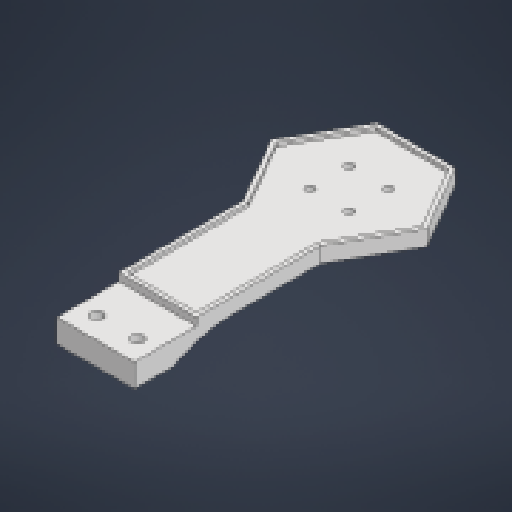
# Autodesk Inventor part: Arm
Saved by Autodesk Inventor 2023 (Build 270158000, 158)
## iProperties
Created: 2023-01-21
Part Number: Arm
Material: Generic
Document SubType Name: Modeling
Designer: Michael
Density: 1 g/cm^3
Appearance: Default
Author: Michael
Autodesk Inventor part; units mm, degrees
ref_plane "YZ Plane" through (0, 0, 0) normal (1, 0, 0) x (0, 1, 0)
ref_plane "XZ Plane" through (0, 0, 0) normal (0, 1, 0) x (-1, 0, 0)
ref_plane "XY Plane" through (0, 0, 0) normal (0, 0, 1) x (1, 0, 0)
sketch "Sketch1" plane through (0, 0, 0) normal (0, 1, 0) x (-1, 0, 0)
  line L0 (0, 0) -> (31.75, 0)
  line L1 (31.75, 0) -> (31.75, -76.2)
  line L2 (31.75, -76.2) -> (0, -76.2)
  line L3 (0, -76.2) -> (0, 0)
  line L4 (31.75, -131.1926) -> (0, -131.1926)
  line L5 (0, -131.1926) -> (-15.875, -103.6963)
  line L6 (-15.875, -103.6963) -> (0, -76.2)
  line L7 (0, -76.2) -> (31.75, -76.2)
  line L8 (31.75, -76.2) -> (47.625, -103.6963)
  line L9 (47.625, -103.6963) -> (31.75, -131.1926)
  line L10 (7.8765, -95.6953) -> (23.876, -95.6953)
  line L11 (23.876, -95.6953) -> (23.876, -111.6948)
  line L12 (23.876, -111.6948) -> (7.8765, -111.6948)
  line L13 (7.8765, -111.6948) -> (7.8765, -95.6953)
  circle A0 centre (23.876, -95.6953) radius 1.6993
  circle A1 centre (23.876, -111.6948) radius 1.6993
  circle A2 centre (7.8765, -111.6948) radius 1.6993
  circle A3 centre (7.8765, -95.6953) radius 1.6993
  point P0 (15.875, -103.6963)
  point P1 (15.875, -76.2)
  point P2 (15.8763, -95.6953)
  point P3 (31.75, -76.2)
  point P4 (0, -76.2)
  dimension "d0" = 31.75
  dimension "d1" = 76.2
  dimension "d65" = 31.75
  dimension "d66" = 15.9995
  dimension "d67" = 15.9995
  dimension "d68" = 8.001
  dimension "d69" = 8.001
  dimension "d70" = 3.3985
  dimension "d71" = 3.3985
  dimension "d72" = 3.3985
  dimension "d73" = 3.3985
  constraints: 28 end point, 5 parallel, 4 centre point, 4 coincident, 3 midpoint, 2 horizontal, 2 perpendicular, 13 other
  measures "d0" distance of L1.end L2.end
  measures "d1" distance of L0.end L1.end
  measures "d65" distance of L6.end L7.end
  measures "d66" distance of L10.start L10.end
  measures "d67" distance of L10.end L11.end
  measures "d68" distance from line of L11 point (15.875, -103.696)
  measures "d69" distance of point (15.876, -95.695) point (15.875, -103.696)
  measures "d70" diameter of A0
  measures "d71" diameter of A1
  measures "d72" diameter of A2
  measures "d73" diameter of A3
extrude "Extrusion1" add sketch "Sketch1" along normal blind 6.35 contours L0 L1 L2 L3 | L2 L8 L9 L4 L5 L6 | L10 A0 L11 A1 L12 A2 L13 A3
sketch "Sketch2" plane through (0, 0, 0) normal (0, -1, 0) x (1, 0, 0)
  line L0 (0, 0) -> (0, -76.2) projected
  line L1 (0, 0) -> (-31.75, 0)
  line L2 (-31.75, 0) -> (-31.75, -31.75)
  line L3 (-31.75, -31.75) -> (0, -31.75)
  line L4 (0, -31.75) -> (0, 0)
  point P0 (0, -127)
  point P1 (0, -31.75)
  dimension "d4" = 31.75
  dimension "d5" = 31.75
  constraints: 8 end point, 2 parallel, 1 horizontal, 1 perpendicular
  measures "d4" distance of L3.end L2.end
  measures "d5" distance of L2.end L1.end
extrude "Extrusion2" add sketch "Sketch2" along normal blind 6.35
fillet "Fillet1" radius 50.8 1 edges at (-15.875, 0, -31.75)
sketch "Sketch4" plane through (0, 6.35, 0) normal (0, 1, 0) x (1, 0, 0)
  circle A0 centre (-7.62, 8.89) radius 2.4765
  line L0 (-31.75, 0) -> (0, 0) projected
  line L1 (0, 0) -> (0, 76.2) projected
  circle A1 centre (-24.13, 8.89) radius 2.4765
  line L2 (-31.75, 76.2) -> (-31.75, 0) projected
  point P0 (0, 127)
  point P1 (-31.75, 127)
  dimension "d11" = 4.953
  dimension "d12" = 8.89
  dimension "d13" = 7.62
  dimension "d14" = 4.953
  dimension "d15" = 8.89
  dimension "d16" = 7.62
  constraints: 2 centre point
  measures "d11" diameter of A0
  measures "d12" distance from line of L0 A0.centre
  measures "d13" distance from line of A0.centre L1
  measures "d14" diameter of A1
  measures "d15" distance from line of L0 A1.centre
  measures "d16" distance from line of L2 A1.centre
extrude "Extrusion4" cut sketch "Sketch4" against normal blind 36.5125
sketch "Sketch7" plane through (0, 6.35, 0) normal (0, 1, 0) x (1, 0, 0)
  arc A0 (20.5419, -92.0874) -> (18.9723, -84.4373) centre (2.0814, -91.8891) ccw projected
  arc A1 (20.2921, -77.3839) -> (18.9723, -84.4373) centre (24.782, -81.8742) ccw projected
  line L0 (20.2921, -77.3839) -> (36.3529, -61.3246) projected
  arc A2 (45.3332, -61.3251) -> (36.3529, -61.3246) centre (40.8428, -65.815) ccw projected
  line L1 (45.3332, -61.3251) -> (71.6731, -87.6679) projected
  arc A3 (67.1824, -98.5077) -> (71.6731, -87.6679) centre (67.1827, -92.1577) ccw projected
  line L2 (67.1824, -98.5077) -> (26.8912, -98.5056) projected
  arc A4 (20.5419, -92.0874) -> (26.8912, -98.5056) centre (26.8916, -92.1556) ccw projected
  circle A5 centre (2.0814, -91.8891) radius 12.2682 projected
  line L3 (71.6717, -113.6942) -> (23.813, -161.5477) projected
  arc A6 (12.9731, -157.057) -> (23.813, -161.5477) centre (19.3231, -157.0573) ccw projected
  line L4 (12.9731, -157.057) -> (12.9757, -109.6932) projected
  arc A7 (14.9079, -105.1323) -> (12.9757, -109.6932) centre (19.3257, -109.6936) ccw projected
  arc A8 (14.9079, -105.1323) -> (15.2755, -104.7661) centre (2.0814, -91.8891) ccw projected
  arc A9 (19.8202, -102.8513) -> (15.2755, -104.7661) centre (19.8199, -109.2013) ccw projected
  line L5 (19.8202, -102.8513) -> (67.1821, -102.8538) projected
  arc A10 (71.6717, -113.6942) -> (67.1821, -102.8538) centre (67.1818, -109.2038) ccw projected
  line L6 (-67.3349, -70.3528) -> (-19.6044, -22.6275) projected
  arc A11 (-8.7645, -27.1173) -> (-19.6044, -22.6275) centre (-15.1145, -27.1179) ccw projected
  line L7 (-8.7645, -27.1173) -> (-8.7605, -74.0286) projected
  arc A12 (-10.7068, -78.604) -> (-8.7605, -74.0286) centre (-15.1105, -74.0291) ccw projected
  arc A13 (-10.7068, -78.604) -> (-11.2559, -79.1554) centre (2.0814, -91.8891) ccw projected
  arc A14 (-15.8389, -81.1204) -> (-11.2559, -79.1554) centre (-15.8487, -74.7704) ccw projected
  line L8 (-15.8389, -81.1204) -> (-62.8352, -81.1932) projected
  arc A15 (-67.3349, -70.3528) -> (-62.8352, -81.1932) centre (-62.845, -74.8432) ccw projected
  line L9 (-41.0097, -122.7457) -> (-67.4831, -96.2695) projected
  arc A16 (-62.9912, -85.4296) -> (-67.4831, -96.2695) centre (-62.9927, -91.7796) ccw projected
  line L10 (-62.9912, -85.4296) -> (-22.7324, -85.439) projected
  arc A17 (-16.3839, -91.8146) -> (-22.7324, -85.439) centre (-22.7338, -91.789) ccw projected
  arc A18 (-16.3839, -91.8146) -> (-14.7078, -99.5763) centre (2.0814, -91.8891) ccw projected
  arc A19 (-15.9916, -106.7102) -> (-14.7078, -99.5763) centre (-20.4814, -102.2198) ccw projected
  line L11 (-15.9916, -106.7102) -> (-32.0295, -122.7462) projected
  arc A20 (-41.0097, -122.7457) -> (-32.0295, -122.7462) centre (-36.5194, -118.2558) ccw projected
  line L12 (-2.2134, -161.5463) -> (-28.5533, -135.2035) projected
  arc A21 (-28.5528, -126.2232) -> (-28.5533, -135.2035) centre (-24.0629, -130.7136) ccw projected
  line L13 (-28.5528, -126.2232) -> (-12.4256, -110.098) projected
  arc A22 (-5.372, -108.7789) -> (-12.4256, -110.098) centre (-7.9357, -114.5884) ccw projected
  arc A23 (-5.372, -108.7789) -> (2.2286, -110.3498) centre (2.0814, -91.8891) ccw projected
  arc A24 (8.6292, -116.7) -> (2.2286, -110.3498) centre (2.2792, -116.6996) ccw projected
  line L14 (8.6292, -116.7) -> (8.627, -157.0567) projected
  arc A25 (-2.2134, -161.5463) -> (8.627, -157.0567) centre (2.277, -157.0564) ccw projected
  arc A26 (9.7706, -75.1005) -> (1.9589, -73.4238) centre (2.0814, -91.8891) ccw projected
  arc A27 (-4.4332, -67.0716) -> (1.9589, -73.4238) centre (1.9168, -67.0739) ccw projected
  line L15 (-4.4332, -67.0716) -> (-4.4185, -26.8971) projected
  arc A28 (6.4218, -22.4095) -> (-4.4185, -26.8971) centre (1.9315, -26.8994) ccw projected
  line L16 (6.4218, -22.4095) -> (32.8767, -48.8673) projected
  arc A29 (32.8763, -57.8475) -> (32.8767, -48.8673) centre (28.3863, -53.3572) ccw projected
  line L17 (32.8763, -57.8475) -> (16.9047, -73.8175) projected
  arc A30 (9.7706, -75.1005) -> (16.9047, -73.8175) centre (12.4148, -69.3272) ccw projected
  line L18 (119.3668, -125.7332) -> (119.3702, -93.9832) projected
  line L19 (119.3702, -93.9832) -> (93.9702, -93.9804) projected
  line L20 (93.9702, -93.9804) -> (0, 0) projected
  line L21 (0, 0) -> (0, 25.4) projected
  line L22 (0, 25.4) -> (-31.75, 25.4) projected
  line L23 (-31.75, 25.4) -> (-31.75, 0) projected
  line L24 (-31.75, 0) -> (-89.804, -58.0477) projected
  line L25 (-89.804, -58.0477) -> (-115.204, -58.0449) projected
  line L26 (-115.204, -58.0449) -> (-115.2074, -89.7949) projected
  line L27 (-115.2074, -89.7949) -> (-89.8074, -89.7977) projected
  line L28 (-89.8074, -89.7977) -> (4.1628, -183.7781) projected
  line L29 (4.1628, -183.7781) -> (4.1628, -209.1781) projected
  line L30 (4.1628, -209.1781) -> (35.9128, -209.1781) projected
  line L31 (35.9128, -209.1781) -> (35.9128, -183.7781) projected
  line L32 (35.9128, -183.7781) -> (93.9668, -125.7304) projected
  line L33 (93.9668, -125.7304) -> (119.3668, -125.7332) projected
  circle A31 centre (102.8594, -101.6014) radius 2.2479 projected
  circle A32 centre (102.8576, -118.1114) radius 2.2479 projected
  circle A33 centre (28.2928, -192.6681) radius 2.2479 projected
  circle A34 centre (11.7828, -192.6681) radius 2.2479 projected
  circle A35 centre (-98.6948, -65.6667) radius 2.2479 projected
  circle A36 centre (-98.6966, -82.1767) radius 2.2479 projected
  circle A37 centre (-7.62, 8.89) radius 2.2479 projected
  circle A38 centre (-24.13, 8.89) radius 2.2479 projected
  line L34 (-31.75, 76.2) -> (-31.75, 0) projected
  line L35 (0, 25.4) -> (-31.75, 25.4)
  line L36 (-31.75, 25.4) -> (-31.75, 0)
  line L37 (-31.75, 0) -> (0, 0)
  line L38 (0, 0) -> (0, 25.4)
  constraints: 8 end point, 2 parallel, 1 horizontal, 1 perpendicular
extrude "Extrusion6" cut sketch "Sketch7" against normal blind 3.175 contours L37 L23 L22 L21
sketch "Sketch8" plane through (0, 6.35, 0) normal (0, 1, 0) x (1, 0, 0)
  circle A0 centre (-7.8765, 95.6953) radius 1.6993 projected
  circle A1 centre (-7.8765, 111.6948) radius 1.6993 projected
  circle A2 centre (-23.876, 111.6948) radius 1.6993 projected
  circle A3 centre (-23.876, 95.6953) radius 1.6993 projected
  line L0 (-31.75, 25.4) -> (0, 25.4) projected
  line L1 (0, 25.4) -> (0, 76.2) projected
  line L2 (0, 76.2) -> (15.875, 103.6963) projected
  line L3 (15.875, 103.6963) -> (0, 131.1926) projected
  line L4 (0, 131.1926) -> (-31.75, 131.1926) projected
  line L5 (-31.75, 131.1926) -> (-47.625, 103.6963) projected
  line L6 (-47.625, 103.6963) -> (-31.75, 76.2) projected
  line L7 (-31.75, 76.2) -> (-31.75, 25.4) projected
  line L8 (-30.0159, 27.1341) -> (-1.7341, 27.1341)
  line L9 (-1.7341, 27.1341) -> (-1.7341, 76.6646)
  line L10 (-1.7341, 76.6646) -> (13.8726, 103.6963)
  line L11 (13.8726, 103.6963) -> (-1.0012, 129.4585)
  line L12 (-1.0012, 129.4585) -> (-30.7488, 129.4585)
  line L13 (-30.7488, 129.4585) -> (-45.6226, 103.6963)
  line L14 (-45.6226, 103.6963) -> (-30.0159, 76.6646)
  line L15 (-30.0159, 76.6646) -> (-30.0159, 27.1341)
  point P0 (0, 0)
  constraints: 16 end point, 7 other
extrude "Extrusion7" cut sketch "Sketch8" against normal blind 1.5875 contours L15 L14 L13 L12 L11 L10 L9 L8
sketch "Sketch9" plane through (-1.7341, 6.35, -27.1341) normal (0, 0, -1) x (-1, 0, 0)
  line L0 (0, 0) -> (28.2818, 0) projected
  line L1 (0, 0) -> (0, -1.5875) projected
  line L2 (0, -1.5875) -> (28.2818, -1.5875) projected
  line L3 (28.2818, 0) -> (28.2818, -1.5875) projected
  line L4 (30.0159, 0) -> (-1.7341, 0) projected
  line L5 (14.1409, 0) -> (14.1409, -1.5875)
  line L6 (21.2148, 0) -> (24.3898, 0)
  line L7 (-1.7341, -3.175) -> (30.0159, -3.175) projected
  line L8 (21.2148, 0) -> (18.0398, 0)
  line L9 (18.0398, 0) -> (18.0398, -1.5875)
  line L10 (24.3898, 0) -> (24.3898, -1.5875)
  line L11 (28.2818, 0) -> (0, 0)
  line L12 (-1.7341, 0) -> (30.0159, 0)
  line L13 (7.067, 0) -> (3.892, 0)
  line L14 (7.067, 0) -> (10.242, 0)
  line L15 (10.242, 0) -> (10.242, -1.5875)
  line L16 (3.892, 0) -> (3.892, -1.5875)
  point P0 (-1.7341, -6.35)
  point P1 (14.1409, -0.7937)
  point P2 (3.892, 0)
  point P3 (3.892, -1.5875)
  point P4 (10.242, 0)
  dimension "d79" = 7.0739
  dimension "d80" = 3.175
  dimension "d82" = 3.175
  constraints: 22 end point, 9 symmetric about line, 4 point on line, 3 midpoint, 2 perpendicular, 1 collinear, 1 horizontal
  measures "d79" horizontal distance of point (14.141, -0.794) L6.start
  measures "d80" distance of L6.start L6.end
  measures "d82" distance of L6.start L8.end
extrude "Extrusion8" add sketch "Sketch9" along normal blind 49.2125 contours L0 L15 L2 L16 | L0 L10 L2 L9
fillet "Fillet2" radius 3.175 2 edges at (-8.8011, 6.35, -76.3466) (-22.9489, 6.35, -76.3466)
fillet "Fillet4" radius 3.175 4 edges at (-45.6226, 5.5562, -103.6963) (13.8726, 5.5562, -103.6963) (-30.7488, 5.5562, -129.4585) (-1.0012, 5.5562, -129.4585)
body "Solid1"
